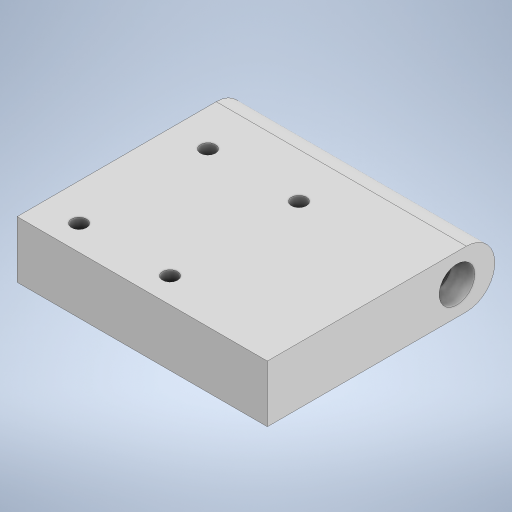
# Autodesk Inventor part: sensor bendor
Saved by Autodesk Inventor 2024.2 (Build 282272000, 272)
## iProperties
Created: 2024-07-10
Part Number: sensor bendor
Material: Generic
Document SubType Name: Modeling
Designer: Tom
Density: 1 g/cm^3
Appearance: Default
Author: Tom
Autodesk Inventor part; units mm, degrees
ref_plane "YZ Plane" through (0, 0, 0) normal (1, 0, 0) x (0, 1, 0)
ref_plane "XZ Plane" through (0, 0, 0) normal (0, 1, 0) x (-1, 0, 0)
ref_plane "XY Plane" through (0, 0, 0) normal (0, 0, 1) x (1, 0, 0)
sketch "Sketch1" plane through (0, 0, 0) normal (0, 1, 0) x (-1, 0, 0)
  line L0 (-16.3555, 0) -> (25.5545, 0)
  line L1 (25.5545, 0) -> (25.5545, -38.1)
  line L2 (25.5545, -38.1) -> (-16.3555, -38.1)
  line L3 (-16.3555, -38.1) -> (-16.3555, 0)
  point P0 (0, 0)
  dimension "d0" = 41.91
  dimension "d1" = 38.1
  constraints: 8 end point, 2 parallel, 1 horizontal, 1 perpendicular
  measures "d0" distance of L0.start L0.end
  measures "d1" distance of L0.end L1.end
extrude "Extrusion1" add sketch "Sketch1" along normal blind 9.525
sketch "Sketch2" plane through (16.3555, 0, 0) normal (1, 0, 0) x (0, 0, -1)
  circle A0 centre (31.75, 4.7625) radius 1.4986
  line L0 (0, 0) -> (38.1, 0) projected
  line L1 (38.1, 0) -> (38.1, 9.525) projected
  dimension "d4" = 2.9972
  dimension "d5" = 4.7625
  dimension "d6" = 6.35
  constraints: 1 centre point
  measures "d4" diameter of A0
  measures "d5" distance from line of L0 A0.centre
  measures "d6" distance from line of L1 A0.centre
extrude "Extrusion2" cut sketch "Sketch2" against normal through all
sketch "Sketch3" plane through (16.3555, 0, 0) normal (1, 0, 0) x (0, 0, -1)
  circle A0 centre (31.75, 4.7625) radius 1.4986 projected
  circle A1 centre (31.75, 4.7625) radius 2.9845
  circle A2 centre (31.75, 4.7625) radius 1.4986
  point P0 (0, 0)
  dimension "d9" = 5.969
  constraints: 2 centre point, 2 coincident, 1 concentric
  measures "d9" diameter of A1
extrude "Extrusion3" cut sketch "Sketch3" against normal blind 3.81
sketch "Sketch4" plane through (0, 9.525, 0) normal (0, 1, 0) x (1, 0, 0)
  line L0 (-19.3894, 4.2047) -> (-4.1494, 4.2047)
  line L1 (-4.1494, 4.2047) -> (-4.1494, 25.7947)
  line L2 (-4.1494, 25.7947) -> (-19.3894, 25.7947)
  line L3 (-19.3894, 25.7947) -> (-19.3894, 4.2047)
  line L4 (16.3555, 38.1) -> (-25.5545, 38.1) projected
  line L5 (-25.5545, 38.1) -> (-25.5545, 0) projected
  circle A0 centre (-19.3894, 4.2047) radius 1.27
  circle A1 centre (-4.1494, 4.2047) radius 1.27
  circle A2 centre (-4.1494, 25.7947) radius 1.27
  circle A3 centre (-19.3894, 25.7947) radius 1.27
  point P0 (0, 0)
  point P1 (-19.3894, 14.9997)
  dimension "d12" = 21.59
  dimension "d14" = 15.24
  dimension "d16" = 2.54
  dimension "d17" = 2.54
  dimension "d20" = 2.54
  constraints: 8 end point, 6 coincident, 4 centre point, 2 parallel, 1 horizontal, 1 midpoint, 1 perpendicular, 2 other
  measures "d12" distance of L2.end L0.start
  measures "d14" distance of L0.start L0.end
  measures "d16" diameter of A0
  measures "d17" diameter of A1
  measures "d20" diameter of A3
extrude "Extrusion4" cut sketch "Sketch4" against normal through all contours L3 A0 L0 | L0 A0 L3 | A1 L1 L0 | L0 L1 A1 | A3 L2 L3 | L3 L2 A3 | A2 L2 L1 | L1 L2 A2
full round fillet "Full Round Fillet1" first side at (9.9315, 9.525, -21.1969) centre faces at (2.3855, 3.175, -38.1) second side at (9.9315, 0, -21.1969)
body "Solid1"
